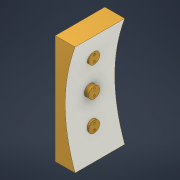
# Autodesk Inventor part: LED Reflector
Saved by Autodesk Inventor 2022 (Build 260153000, 153)
## iProperties
Created: 2021-08-06
Part Number: LED Reflector
Material: Generic
Document SubType Name: Modeling
Designer: sidsa
Density: 1 g/cm^3
Appearance: Brass - Satin
Author: sidsa
Autodesk Inventor part; units mm, degrees
ref_plane "YZ Plane" through (0, 0, 0) normal (1, 0, 0) x (0, 1, 0)
ref_plane "XZ Plane" through (0, 0, 0) normal (0, 1, 0) x (-1, 0, 0)
ref_plane "Work Plane1" through (6.35, -34.925, 15.875) normal (0, 0, 1) x (1, 0, 0)
sketch "Sketch3" plane through (6.35, -34.925, 15.875) normal (0, 0, 1) x (1, 0, 0)
  line L0 (1.5875, 69.85) -> (1.5875, 0) projected
  line L1 (14.2875, 0) -> (1.5875, 34.925) construction
  line L2 (1.5875, 34.925) -> (14.2875, 69.85) construction
  spline S0 degree 2 poles (14.2875, 0) (1.5875, 34.925) (14.2875, 69.85) knots 1 1 1 2 2 2
  line L3 (1.5875, 69.85) -> (14.2875, 69.85)
  line L4 (14.2875, 0) -> (1.5875, 0)
  point P0 (-6.35, 34.925)
  dimension "d9" = 12.7
  dimension "d10" = 12.7
  constraints: 4 end point, 1 midpoint, 1 parallel, 4 other
  measures "d9" distance of L0.start L2.end
  measures "d10" distance of L0.end L1.start
extrude "Extrusion3" add sketch "Sketch3" against normal blind 31.75
sketch "Sketch4" plane through (7.9375, -34.925, 15.875) normal (-1, 0, 0) x (0, 0, 1)
  line L0 (0, 69.85) -> (0, 0) projected
  line L1 (0, 69.85) -> (-31.75, 69.85) projected
  line L2 (-31.75, 0) -> (-31.75, 69.85) projected
  line L3 (0, 0) -> (-31.75, 0) projected
  line L4 (0, 0) -> (-31.75, 0) construction
  line L5 (-15.875, 0) -> (-15.875, 69.85) construction
  line L6 (0, 69.85) -> (-31.75, 69.85) construction
  circle A0 centre (-15.875, 33.02) radius 0.635
  circle A1 centre (-15.875, 36.83) radius 0.635
  circle A2 centre (-15.875, 34.925) radius 3.6195
  circle A3 centre (-15.875, 52.07) radius 0.635
  circle A4 centre (-15.875, 55.88) radius 0.635
  circle A5 centre (-15.875, 53.975) radius 3.6195
  circle A6 centre (-15.875, 13.97) radius 0.635
  circle A7 centre (-15.875, 17.78) radius 0.635
  circle A8 centre (-15.875, 15.875) radius 3.6195
  circle A9 centre (-15.875, 33.02) radius 0.635
  circle A10 centre (-15.875, 36.83) radius 0.635
  circle A11 centre (-15.875, 34.925) radius 3.6195
  dimension "d13" = 1.27
  dimension "d14" = 1.27
  dimension "d15" = 1.905
  dimension "d16" = 1.905
  dimension "d17" = 7.239
  dimension "d20" = 19.05
  dimension "d23" = 19.05
  constraints: 12 centre point, 4 coincident, 2 end point, 2 midpoint, 2 point on line, 2 vertical, 21 other
  measures "d13" diameter of A0
  measures "d14" diameter of A1
  measures "d15" distance of point (-15.875, 34.925) A0.centre
  measures "d16" distance of point (-15.875, 34.925) A1.centre
  measures "d17" diameter of A2
  measures "d20" distance of point (-15.875, 34.925) point (-15.875, 53.975)
  measures "d23" distance of point (-15.875, 34.925) point (-15.875, 15.875)
extrude "Extrusion4" add sketch "Sketch4" against normal blind 9.017 contours A2 | A5 | A8
sketch "Sketch5" plane through (16.9545, -34.925, 15.875) normal (1, 0, 0) x (0, 0, -1)
  arc A0 (15.3692, 57.559) -> (16.3808, 57.559) centre (15.875, 53.975) ccw projected
  circle A1 centre (15.875, 55.88) radius 0.635 projected
  circle A2 centre (15.875, 52.07) radius 0.635 projected
  circle A3 centre (15.875, 34.925) radius 3.6195 projected
  circle A4 centre (15.875, 33.02) radius 0.635 projected
  circle A5 centre (15.875, 36.83) radius 0.635 projected
  arc A6 (16.3808, 12.291) -> (15.3692, 12.291) centre (15.875, 15.875) ccw projected
  circle A7 centre (15.875, 17.78) radius 0.635 projected
  circle A8 centre (15.875, 13.97) radius 0.635 projected
  constraints: 2 horizontal alignment
extrude "Extrusion5" cut sketch "Sketch5" against normal blind 9.017 contours A1 | A2 | A4 | A5 | A7 | A8
body "Solid1"
